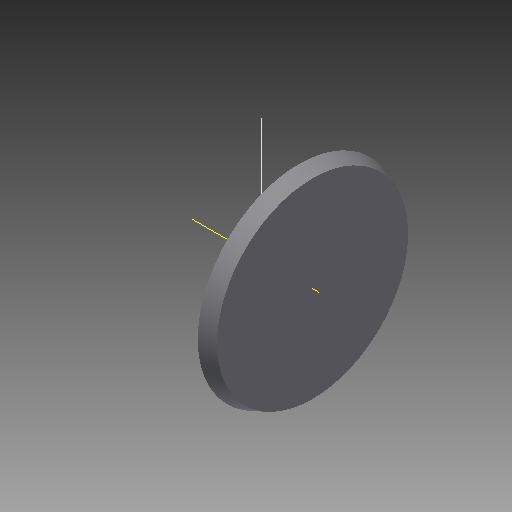
# Autodesk Inventor part: bevelgear_wheel2
Saved by Autodesk Inventor 2019 (Build 230136000, 136)
## iProperties
Shininess: 64.0
Angle Display Precision: 2
Document Length Units: 11269
Document Angle Units: 11279
Document Time Units: 11290
Document Mass Units: 11283
Document Length Units Precision: 3
Document Angle Units Precision: 2
Created: 2005-03-17
Part Number: bevelgear_wheel2
Document SubType Name: Modeling
Designer: Miroslav Petele
Density: 1 g/cm^3
Material: Generic
Appearance: Default
Density: 0.0
Volumn: 0.0
Area: 0.0
PropertySet Name: Model Information
Control State: 0
Master: False
Checked Out: False
Author: Miroslav Petele
Autodesk Inventor part; units mm, degrees
ref_plane "YZ Plane" through (0, 0, 0) normal (1, 0, 0) x (0, 1, 0)
ref_plane "XZ Plane" through (0, 0, 0) normal (0, 1, 0) x (-1, 0, 0)
ref_plane "Work Plane1" through (0, 0, -10) normal (-1, 0, 0) x (0, -1, 0)
sketch "Sketch1" plane through (0, 0, 0) normal (0, 0, 1) x (1, 0, 0)
  line L0 (-21.83974, 0) -> (131.038441, 0)
  line L1 (0, 0) -> (11.555806, 28.889516) construction
  line L2 (93.359081, 201.02678) -> (142.712708, 307.298186)
  line L3 (93.359081, 201.02678) -> (98.847306, 198.83149)
  line L4 (98.847306, 198.83149) -> (98.847306, 0)
  line L5 (142.712708, 307.298186) -> (161.235818, 299.888942)
  line L6 (161.235818, 299.888942) -> (161.235818, 0)
  dimension "delta" = 68.1986
  dimension "hxe" = 19.95
  dimension "hxi" = 5.911
  dimension "hfe" = 18.37774
  dimension "hfi" = 12.02226
  dimension "Ri" = 221.32137
  dimension "b" = 117
  constraints: 12 end point, 4 perpendicular, 2 point on line
  measures "delta" angle of L0 L1
  measures "hxe" distance of L2.end L5.end
  measures "hxi" distance of L2.start L3.end
  measures "hfe" distance from line of L1 L2.end
  measures "hfi" distance from line of L1 L2.start
  measures "Ri" distance from line of L1.start L3
  measures "b" distance between parallel lines of L5 L3
sketch "Sketch1 outline for Revolution1" plane through (0, 0, 0) normal (0, 0, 1) x (1, 0, 0)
  line L0 (98.847306, 198.83149) -> (98.847306, 0)
  line L1 (93.359081, 201.02678) -> (98.847306, 198.83149)
  line L2 (142.712708, 307.298186) -> (93.359081, 201.02678)
  line L3 (161.235818, 299.888942) -> (142.712708, 307.298186)
  line L4 (161.235818, 0) -> (161.235818, 299.888942)
  line L5 (98.847306, 0) -> (161.235818, 0)
revolve "Revolution1" add sketch "Sketch1 outline for Revolution1" angle 360 about axis through (-10, 0, 0) along (1, 0, 0)
sketch "Sketch2" plane through (0, 0, 0) normal (0, 0, 1) x (1, 0, 0)
  line L0 (-20.687045, 0) -> (124.12227, 0)
  line L1 (0, 0) -> (11.984241, 29.960604) construction
  line L2 (93.359081, 201.02678) -> (142.712708, 307.298186)
  line L3 (93.359081, 201.02678) -> (77.202995, 207.489214)
  line L4 (142.712708, 307.298186) -> (118.015819, 317.176941)
  line L5 (118.015819, 317.176941) -> (77.202995, 207.489214)
  dimension "hae" = 8.22162
  dimension "hai" = 5.37838
  dimension "d10" = 68.1986
  constraints: 8 end point, 1 parallel, 1 perpendicular
  measures "hae" distance from line of L1 L4.end
  measures "hai" distance from line of L1 L3.end
  measures "d10" angle of L0 L1
revolve "Revolution2" add sketch "Sketch2" angle 360 about axis through (-10, 0, 0) along (1, 0, 0)
equation "\"delta\" = MC_delta2"
equation "\"hxe\" = MC_hxe2 + MC_hae2 - MC_h2E"
equation "\"hxi\" = MC_hxi2 + MC_hai2 - MC_h2A"
equation "\"hfe\" = MC_h2E - MC_hae2"
equation "\"hfi\" = MC_h2A - MC_hai2"
equation "\"Ri\" = MC_Ri"
equation "\"b\" = MC_b"
equation "\"hae\" = MC_hae2"
equation "\"hai\" = MC_hai2"
equation "\"d10\" = delta"
equation "\"SumDelta\" = MC_deltasum"
equation "\"MC_deltasum\" = 90deg"
equation "\"MC_b\" = 117"
equation "\"MC_Ri\" = 221.32137"
equation "\"MC_alfa\" = 20deg"
equation "\"MC_delta1\" = 21.801409deg"
equation "\"MC_hae1\" = 15.95962"
equation "\"MC_hxe1\" = 23.93975"
equation "\"MC_hai1\" = 10.44038"
equation "\"MC_hxi1\" = 11.79625"
equation "\"MC_delta2\" = 68.1986deg"
equation "\"MC_hae2\" = 8.22162"
equation "\"MC_hxe2\" = 38.32774"
equation "\"MC_hai2\" = 5.37838"
equation "\"MC_hxi2\" = 17.93326"
equation "\"MC_Ang1A\" = 203.543093deg"
equation "\"MC_Ang1B\" = 190.397416deg"
equation "\"MC_Ang1C\" = 180deg"
equation "\"MC_Ang1D\" = 171.570572deg"
equation "\"MC_Ang1E\" = 164.598698deg"
equation "\"MC_Ang2A\" = 170.582763deg"
equation "\"MC_Ang2B\" = 175.841034deg"
equation "\"MC_Ang2C\" = 180deg"
equation "\"MC_Ang2D\" = 183.371771deg"
equation "\"MC_Ang2E\" = 186.160521deg"
equation "\"MC_h1A\" = 17.40064"
equation "\"MC_h1B\" = 19.70032"
equation "\"MC_h1C\" = 22"
equation "\"MC_h1D\" = 24.29968"
equation "\"MC_h1E\" = 26.59936"
equation "\"MC_h2A\" = 17.40064"
equation "\"MC_h2B\" = 19.70032"
equation "\"MC_h2C\" = 22"
equation "\"MC_h2D\" = 24.29968"
equation "\"MC_h2E\" = 26.59936"
equation "\"MC_Rz1A\" = 82.19669"
equation "\"MC_Rz1B\" = 93.05987"
equation "\"MC_Rz1C\" = 103.92305"
equation "\"MC_Rz1D\" = 114.78623"
equation "\"MC_Rz1E\" = 125.6494"
equation "\"MC_Rz2A\" = 205.49173"
equation "\"MC_Rz2B\" = 232.64968"
equation "\"MC_Rz2C\" = 259.80762"
equation "\"MC_Rz2D\" = 286.96556"
equation "\"MC_Rz2E\" = 314.12351"
equation "\"MC_Sa1A\" = 2.90562"
equation "\"MC_Sa1B\" = 3.28962"
equation "\"MC_Sa1C\" = 3.67363"
equation "\"MC_Sa1D\" = 4.05764"
equation "\"MC_Sa1E\" = 4.44165"
equation "\"MC_Sa2A\" = 4.42236"
equation "\"MC_Sa2B\" = 5.00682"
equation "\"MC_Sa2C\" = 5.59128"
equation "\"MC_Sa2D\" = 6.17574"
equation "\"MC_Sa2E\" = 6.7602"
equation "\"MC_tx1A\" = 13.29713"
equation "\"MC_tx1B\" = 15.05449"
equation "\"MC_tx1C\" = 16.81185"
equation "\"MC_tx1D\" = 18.56921"
equation "\"MC_tx1E\" = 20.32657"
equation "\"MC_tx2A\" = 10.0867"
equation "\"MC_tx2B\" = 11.41977"
equation "\"MC_tx2C\" = 12.75284"
equation "\"MC_tx2D\" = 14.0859"
equation "\"MC_tx2E\" = 15.41897"
equation "\"MC_bD\" = 29.25"
equation "\"MC_bC\" = 58.5"
equation "\"MC_bB\" = 87.75"
equation "\"MC_bA\" = 119.34"
equation "\"MC_mx1A\" = 7.47431"
equation "\"MC_mx1B\" = 8.46212"
equation "\"MC_mx1C\" = 9.44993"
equation "\"MC_mx1D\" = 10.43775"
equation "\"MC_mx1E\" = 11.42556"
equation "\"MC_mx2A\" = 7.05073"
equation "\"MC_mx2B\" = 7.98256"
equation "\"MC_mx2C\" = 8.91439"
equation "\"MC_mx2D\" = 9.84622"
equation "\"MC_mx2E\" = 10.77805"
body "Solid1"
